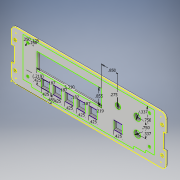
# Autodesk Inventor part: Front Pannel
Saved by Autodesk Inventor 2019 (Build 230136000, 136)
## iProperties
Created: 2020-09-01
Part Number: Front Pannel
Material: Generic
Document SubType Name: Modeling
Designer: johnh
Density: 1 g/cm^3
Appearance: Default
Author: johnh
Autodesk Inventor part; units mm, degrees
ref_plane "YZ Plane" through (0, 0, 0) normal (1, 0, 0) x (0, 1, 0)
ref_plane "XZ Plane" through (0, 0, 0) normal (0, 1, 0) x (-1, 0, 0)
ref_plane "XY Plane" through (0, 0, 0) normal (0, 0, 1) x (1, 0, 0)
sketch "Sketch1" plane through (0, 0, 0) normal (0, 0, 1) x (1, 0, 0)
  line L0 (0, 0) -> (201.5998, 0)
  line L1 (201.5998, 0) -> (201.5998, 63.754)
  line L2 (201.5998, 63.754) -> (0, 63.754)
  line L3 (0, 63.754) -> (0, 0)
  line L4 (0, 41.8592) -> (3.7465, 41.8592)
  line L5 (3.7465, 41.8592) -> (3.7465, 21.8948)
  line L6 (3.7465, 21.8948) -> (0, 21.8948)
  line L7 (0, 21.8948) -> (0, 41.8592)
  line L8 (201.5998, 41.8592) -> (197.8533, 41.8592)
  line L9 (197.8533, 41.8592) -> (197.8533, 21.8948)
  line L10 (197.8533, 21.8948) -> (201.5998, 21.8948)
  line L11 (201.5998, 21.8948) -> (201.5998, 41.8592)
  circle A0 centre (5.0546, 49.1744) radius 1.9558
  circle A1 centre (5.0546, 14.5796) radius 1.9558
  circle A2 centre (196.5452, 14.5796) radius 1.9558
  circle A3 centre (196.5452, 49.1744) radius 1.9558
  dimension "d0" = 201.5998
  dimension "d1" = 63.754
  dimension "d2" = 3.7465
  dimension "d3" = 19.9644
  dimension "d4" = 21.8948
  dimension "d5" = 3.7465
  dimension "d6" = 3.9116
  dimension "d7" = 12.6238
  dimension "d8" = 3.0988
  dimension "d9" = 3.9116
  dimension "d10" = 12.6238
  dimension "d11" = 3.0988
  dimension "d12" = 3.9116
  dimension "d13" = 3.0988
  constraints: 24 end point, 6 parallel, 4 centre point, 3 horizontal, 3 perpendicular, 2 point on line
  measures "d0" distance of L2.end L1.end
  measures "d1" distance of L1.end L0.end
  measures "d2" distance of L4.start L4.end
  measures "d3" distance of L4.end L5.end
  measures "d4" distance between parallel lines of L2 L4
  measures "d5" distance of L8.start L8.end
  measures "d6" diameter of A0
  measures "d7" distance edge to line of A0 L2
  measures "d8" distance edge to line of A0 L3
  measures "d9" diameter of A1
  measures "d10" distance edge to line of A1 L0
  measures "d11" distance edge to line of A1 L3
  measures "d12" diameter of A2
  measures "d13" distance edge to line of A2 L1
extrude "Extrusion1" add sketch "Sketch1" along normal blind 1.8796 contours L3 L6 L5 L4 L2 L1 L8 L9 L10 L0
fillet "Fillet1" radius 6.35 4 edges at (201.5998, 63.754, 0.9398) (201.5998, 0, 0.9398) (0, 63.754, 0.9398) (0, 0, 0.9398)
sketch "Sketch2" plane through (0, 0, 1.8796) normal (0, 0, 1) x (1, 0, 0)
  arc A0 (0, 6.35) -> (6.35, 0) centre (6.35, 6.35) ccw projected
  line L0 (6.35, 0) -> (195.2498, 0) projected
  arc A1 (195.2498, 0) -> (201.5998, 6.35) centre (195.2498, 6.35) ccw projected
  line L1 (201.5998, 6.35) -> (201.5998, 21.8948) projected
  line L2 (201.5998, 21.8948) -> (197.8533, 21.8948) projected
  line L3 (197.8533, 21.8948) -> (197.8533, 41.8592) projected
  line L4 (197.8533, 41.8592) -> (201.5998, 41.8592) projected
  line L5 (201.5998, 41.8592) -> (201.5998, 57.404) projected
  arc A2 (201.5998, 57.404) -> (195.2498, 63.754) centre (195.2498, 57.404) ccw projected
  line L6 (195.2498, 63.754) -> (6.35, 63.754) projected
  arc A3 (6.35, 63.754) -> (0, 57.404) centre (6.35, 57.404) ccw projected
  line L7 (0, 57.404) -> (0, 41.8592) projected
  line L8 (0, 41.8592) -> (3.7465, 41.8592) projected
  line L9 (3.7465, 41.8592) -> (3.7465, 21.8948) projected
  line L10 (3.7465, 21.8948) -> (0, 21.8948) projected
  line L11 (0, 21.8948) -> (0, 6.35) projected
  circle A4 centre (196.5452, 49.1744) radius 1.9558 projected
  circle A5 centre (196.5452, 14.5796) radius 1.9558 projected
  circle A6 centre (5.0546, 14.5796) radius 1.9558 projected
  circle A7 centre (5.0546, 49.1744) radius 1.9558 projected
  line L12 (15.0622, 60.5663) -> (186.5122, 60.5663)
  line L13 (186.5122, 60.5663) -> (186.5122, 9.7663)
  line L14 (15.0622, 9.7663) -> (15.0622, 60.5663)
  line L15 (175.0822, 9.7663) -> (175.0822, 6.5913)
  line L16 (26.4922, 6.5913) -> (26.4922, 9.7663)
  line L17 (159.5247, 6.5913) -> (159.5247, 3.4163)
  line L18 (159.5247, 3.4163) -> (42.0497, 3.4163)
  line L19 (42.0497, 3.4163) -> (42.0497, 6.5913)
  circle A8 centre (21.4122, 54.2163) radius 1.5875
  circle A9 centre (21.4122, 16.129) radius 1.5875
  circle A10 centre (180.1622, 16.129) radius 1.5875
  circle A11 centre (180.1622, 54.229) radius 1.5875
  line L20 (33.3756, 50.5714) -> (117.4496, 50.5714)
  line L21 (117.4496, 50.5714) -> (117.4496, 28.8544)
  line L22 (117.4496, 28.8544) -> (33.3756, 28.8544)
  line L23 (33.3756, 28.8544) -> (33.3756, 50.5714)
  line L24 (38.9255, 23.114) -> (49.7205, 23.114)
  line L25 (49.7205, 23.114) -> (49.7205, 12.319)
  line L26 (49.7205, 12.319) -> (38.9255, 12.319)
  line L27 (38.9255, 12.319) -> (38.9255, 23.114)
  line L28 (54.4576, 23.114) -> (65.2526, 23.114)
  line L29 (65.2526, 23.114) -> (65.2526, 12.319)
  line L30 (65.2526, 12.319) -> (54.4576, 12.319)
  line L31 (54.4576, 12.319) -> (54.4576, 23.114)
  line L32 (70.0024, 23.114) -> (80.7974, 23.114)
  line L33 (80.7974, 23.114) -> (80.7974, 12.319)
  line L34 (80.7974, 12.319) -> (70.0024, 12.319)
  line L35 (70.0024, 12.319) -> (70.0024, 23.114)
  line L36 (85.5472, 23.114) -> (96.3422, 23.114)
  line L37 (96.3422, 23.114) -> (96.3422, 12.319)
  line L38 (96.3422, 12.319) -> (85.5472, 12.319)
  line L39 (85.5472, 12.319) -> (85.5472, 23.114)
  line L40 (101.092, 23.114) -> (111.887, 23.114)
  line L41 (111.887, 23.114) -> (111.887, 12.319)
  line L42 (111.887, 12.319) -> (101.092, 12.319)
  line L43 (101.092, 12.319) -> (101.092, 23.114)
  line L44 (133.6421, 23.114) -> (144.4371, 23.114)
  line L45 (144.4371, 23.114) -> (144.4371, 12.319)
  line L46 (144.4371, 12.319) -> (133.6421, 12.319)
  line L47 (133.6421, 12.319) -> (133.6421, 23.114)
  line L48 (175.0822, 9.7663) -> (186.5122, 9.7663)
  line L49 (26.4922, 9.7663) -> (15.0622, 9.7663)
  line L50 (26.4922, 6.5913) -> (42.0497, 6.5913)
  line L51 (159.5247, 6.5913) -> (175.0822, 6.5913)
  circle A12 centre (164.17, 41.5163) radius 4.2799
  circle A13 centre (164.17, 22.4663) radius 4.2799
  circle A14 centre (139.0396, 41.5163) radius 3.4925
  point P0 (0, 0)
  dimension "d30" = 3.175
  dimension "d31" = 6.35
  dimension "d32" = 6.35
  dimension "d42" = 84.074
  dimension "d43" = 21.717
  dimension "d72" = 10.795
  dimension "d73" = 10.795
  dimension "d74" = 10.795
  dimension "d75" = 10.795
  dimension "d76" = 10.795
  dimension "d77" = 10.795
  dimension "d78" = 10.795
  dimension "d79" = 4.7371
  dimension "d80" = 4.7498
  dimension "d81" = 4.7498
  dimension "d82" = 4.7498
  dimension "d83" = 5.5626
  dimension "d84" = 5.5499
  dimension "d85" = 12.319
  dimension "d86" = 8.5598
  dimension "d87" = 8.5598
  dimension "d88" = 19.05
  dimension "d89" = 19.05
  dimension "d90" = 6.985
  dimension "d91" = 21.59
  constraints: 80 end point, 19 equal length, 10 horizontal, 10 point on line, 8 perpendicular, 7 centre point
  measures "d30" diameter of A8
  measures "d31" distance from line of L12 A8.centre
  measures "d32" distance from line of A8.centre L14
  measures "d42" distance of L21.end L22.end
  measures "d43" distance of L20.end L21.end
  measures "d72" distance of L25.end L26.end
  measures "d73" distance of L24.end L25.end
  measures "d74" distance of L29.end L30.end
  measures "d75" distance of L33.end L34.end
  measures "d76" distance of L37.end L38.end
  measures "d77" distance of L41.end L42.end
  measures "d78" distance of L45.end L46.end
  measures "d79" distance between parallel lines of L31 L25
  measures "d80" distance between parallel lines of L35 L29
  measures "d81" distance between parallel lines of L39 L33
  measures "d82" distance between parallel lines of L43 L37
  measures "d83" distance between parallel lines of L21 L41
  measures "d84" distance between parallel lines of L23 L27
  measures "d85" distance between parallel lines of L0 L26
  measures "d86" diameter of A12
  measures "d87" diameter of A13
  measures "d88" distance of A12.centre A13.centre
  measures "d89" distance from line of A12.centre L12
  measures "d90" diameter of A14
  measures "d91" distance from line of A14.centre L21
extrude "Extrusion2" cut sketch "Sketch2" against normal blind 1.8796 contours A8 | A9 | A10 | A11 | L20 L21 L22 L23 | L24 L25 L26 L27 | L28 L29 L30 L31 | L32 L33 L34 L35 | L36 L37 L38 L39 | L40 L41 L42 L43 | L44 L45 L46 L47 | A12 | A13 | A14
extrude "Extrusion3" add sketch "Sketch2" against normal blind 3.7592 contours L12 L13 L48 L15 L51 L17 L18 L19 L50 L16 L49 L14
body "Solid1"
